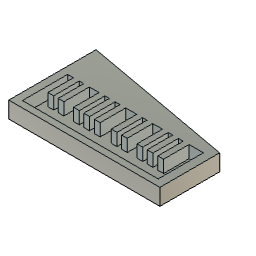
pianoooooo (Autodesk Fusion 360 design; units mm, degrees)
Autodesk Fusion 360 part; units mm, degrees
sketch "草图1" plane through (0, 0, 0) normal (0, 0, 1) x (1, 0, 0)
  line L0 (-83.7376, 48.3346) -> (-83.7376, -57.8018)
  line L1 (100, -57.8018) -> (-83.7376, -57.8018)
  line L2 (99.9425, 14.822) -> (-83.7376, 48.3346)
  line L3 (99.9425, 14.822) -> (99.9425, -57.8018)
  line L4 (-75.3044, 2.9706) -> (90.6956, 2.9706)
  line L5 (90.6956, 2.9706) -> (90.6956, -51.4889)
  line L6 (90.6956, -51.4889) -> (-75.3044, -51.4889)
  line L7 (-75.3044, -51.4889) -> (-75.3044, 2.9706)
  dimension "d1" = 166
  constraint vertical L0
  constraint perpendicular L0 L1
  constraint vertical L3
  constraint horizontal L4
  constraint vertical L5
  constraint horizontal L6
  constraint vertical L7
  measures "d1" distance of L4.start L4.end
extrude "拉伸1" add sketch "草图1" along normal blind 20 contours L0 L1 L2 L3 | L4 L5 L6 L7
sketch "草图2" plane through (0, 0, 20) normal (0, 0, 1) x (-1, 0, 0)
  line L0 (83.7376, -48.3346) -> (83.7376, 57.8018)
  line L1 (83.7376, 57.8018) -> (-99.9425, 57.8018)
  line L2 (-99.9425, 57.8018) -> (-99.9425, -14.822)
  line L3 (-99.9425, -14.822) -> (83.7376, -48.3346)
  line L4 (75, -5) -> (-90, -5)
  line L5 (-90, -5) -> (-90, 50)
  line L6 (-90, 50) -> (75, 50)
  line L7 (75, 50) -> (75, -5)
  constraint horizontal L4
  constraint vertical L5
  constraint horizontal L6
  constraint vertical L7
extrude "拉伸2" cut sketch "草图2" against normal blind 15 contours L4 L5 L6 L7
sketch "草图3" plane through (0, 0, 20) normal (0, 0, 1) x (-1, 0, 0)
  line L0 (-90, -5) -> (-90, 50)
  line L1 (-90, 50) -> (75, 50)
  line L2 (75, 50) -> (75, -5)
  line L3 (75, -5) -> (-90, -5)
  line L4 (83.7376, -48.3346) -> (83.7376, 57.8018)
  line L5 (83.7376, 57.8018) -> (-99.9425, 57.8018)
  line L6 (-99.9425, 57.8018) -> (-99.9425, -14.822)
  line L7 (-99.9425, -14.822) -> (83.7376, -48.3346)
  line L8 (67.985, -5) -> (60.985, -5)
  line L9 (60.985, -5) -> (60.985, 26)
  line L10 (60.985, 26) -> (67.985, 26)
  line L11 (67.985, 26) -> (67.985, -5)
  line L12 (67.985, -5) -> (60.985, -5)
  line L13 (67.985, 26) -> (67.985, -5)
  line L14 (60.985, 26) -> (67.985, 26)
  line L15 (60.985, -5) -> (60.985, 26)
  line L16 (55.5549, 26) -> (55.5549, -5)
  line L17 (55.5549, -5) -> (48.5549, -5)
  line L18 (48.5549, -5) -> (48.5549, 26)
  line L19 (48.5549, 26) -> (55.5549, 26)
  line L20 (55.5549, 26) -> (55.5549, -5)
  line L21 (48.5549, 26) -> (55.5549, 26)
  line L22 (48.5549, -5) -> (48.5549, 26)
  line L23 (55.5549, -5) -> (48.5549, -5)
  line L24 (36.7829, -5) -> (29.7829, -5)
  line L25 (36.7829, 26) -> (36.7829, -5)
  line L26 (29.7829, 26) -> (36.7829, 26)
  line L27 (29.7829, -5) -> (29.7829, 26)
  line L28 (24.3528, 26) -> (24.3528, -5)
  line L29 (17.3528, 26) -> (24.3528, 26)
  line L30 (17.3528, -5) -> (17.3528, 26)
  line L31 (24.3528, -5) -> (17.3528, -5)
  line L32 (11.4154, 26) -> (11.4154, -5)
  line L33 (4.4154, -5) -> (4.4154, 26)
  line L34 (11.4154, -5) -> (4.4154, -5)
  line L35 (4.4154, 26) -> (11.4154, 26)
  line L36 (-52.6472, -5) -> (-59.6472, -5)
  line L37 (-21.4451, 26) -> (-21.4451, -5)
  line L38 (-9.015, -5) -> (-16.015, -5)
  line L39 (-28.4451, 26) -> (-21.4451, 26)
  line L40 (-28.4451, 26) -> (-21.4451, 26)
  line L41 (-40.2171, 26) -> (-40.2171, -5)
  line L42 (-40.2171, -5) -> (-47.2171, -5)
  line L43 (-72.5846, -5) -> (-72.5846, 26)
  line L44 (-47.2171, 26) -> (-40.2171, 26)
  line L45 (-47.2171, -5) -> (-47.2171, 26)
  line L46 (-52.6472, 26) -> (-52.6472, -5)
  line L47 (-65.5846, 26) -> (-65.5846, -5)
  line L48 (-9.015, 26) -> (-9.015, -5)
  line L49 (-16.015, 26) -> (-9.015, 26)
  line L50 (-21.4451, -5) -> (-28.4451, -5)
  line L51 (-28.4451, -5) -> (-28.4451, 26)
  line L52 (-16.015, -5) -> (-16.015, 26)
  line L53 (-28.4451, -5) -> (-28.4451, 26)
  line L54 (-9.015, -5) -> (-16.015, -5)
  line L55 (-16.015, 26) -> (-9.015, 26)
  line L56 (-72.5846, 26) -> (-65.5846, 26)
  line L57 (-65.5846, -5) -> (-72.5846, -5)
  line L58 (-21.4451, 26) -> (-21.4451, -5)
  line L59 (-9.015, 26) -> (-9.015, -5)
  line L60 (-21.4451, -5) -> (-28.4451, -5)
  line L61 (-59.6472, 26) -> (-52.6472, 26)
  line L62 (-59.6472, -5) -> (-59.6472, 26)
  line L63 (-16.015, -5) -> (-16.015, 26)
  line L64 (-82.7432, 26.3749) -> (-82.7432, -4.6251)
  line L65 (-89.7432, 26.3749) -> (-82.7432, 26.3749)
  line L66 (-89.7432, -4.6251) -> (-89.7432, 26.3749)
  line L67 (-82.9307, -4.8125) -> (-89.9307, -4.8125)
  point P0 (-77, 0)
  dimension "d6" = 7
  dimension "d7" = 31
  dimension "d8" = 7
  dimension "d9" = 31
  dimension "d10" = 7
  dimension "d11" = 31
  dimension "d12" = 7
  dimension "d13" = 31
  dimension "d14" = 7
  dimension "d15" = 31
  dimension "d16" = 31
  dimension "d17" = 7
  dimension "d18" = 31
  dimension "d19" = 7
  dimension "d22" = -77
  dimension "d23" = 0
  dimension "d24" = 7
  dimension "d25" = 31
  dimension "d26" = 7
  constraint horizontal L8
  constraint vertical L9
  constraint horizontal L10
  constraint vertical L11
  constraint coincident L3 L8.start
  constraint horizontal L12
  constraint vertical L15
  constraint horizontal L14
  constraint vertical L13
  constraint horizontal L17
  constraint vertical L18
  constraint horizontal L19
  constraint vertical L16
  constraint horizontal L23
  constraint vertical L22
  constraint horizontal L21
  constraint vertical L20
  constraint horizontal L24
  constraint vertical L27
  constraint horizontal L26
  constraint vertical L25
  constraint horizontal L29
  constraint vertical L28
  constraint horizontal L31
  constraint vertical L30
  constraint horizontal L35
  constraint vertical L32
  constraint horizontal L34
  constraint vertical L33
  constraint vertical L66
  constraint horizontal L65
  constraint vertical L64
  constraint horizontal L67
  measures "d6" distance of L8.start L8.end
  measures "d7" distance of L8.start L10.end
  measures "d8" distance of L8.start L8.end
  measures "d9" distance of L8.start L10.end
  measures "d10" distance of L17.end L16.end
  measures "d11" distance of L16.start L16.end
  measures "d12" distance of L17.end L16.end
  measures "d13" distance of L16.start L16.end
  measures "d14" distance of L24.start L24.end
  measures "d15" distance of L25.start L24.start
  measures "d16" distance of L28.end L28.start
  measures "d17" distance of L30.start L28.end
  measures "d18" distance of L32.end L32.start
  measures "d19" distance of L32.end L33.start
  measures "d24" distance of L64.end L66.start
  measures "d25" distance of L64.end L64.start
  measures "d26" distance of L67.end L67.start
extrude "拉伸3" add sketch "草图3" against normal blind 15 contours L3 L43 L47 L56 L57 | L3 L36 L46 L61 L62 | L3 L8 L9 L10 L11 L12 L13 L14 L15 | L3 L41 L42 L44 L45 | L3 L16 L17 L18 L19 L20 L21 L22 L23 | L3 L37 L39 L40 L50 L51 L53 L58 L60 | L3 L24 L25 L26 L27 | L3 L38 L48 L49 L52 L54 L55 L59 L63 | L3 L28 L29 L30 L31 | L3 L32 L33 L34 L35
sketch "草图4" plane through (0, 0, 20) normal (0, 0, 1) x (-1, 0, 0)
  line L0 (-90, -5) -> (-90, 50)
  line L1 (-90, 50) -> (75, 50)
  line L2 (75, 50) -> (75, -5)
  line L3 (75, -5) -> (67.985, -5)
  line L4 (67.985, -5) -> (67.985, 26)
  line L5 (67.985, 26) -> (60.985, 26)
  line L6 (60.985, 26) -> (60.985, -5)
  line L7 (60.985, -5) -> (55.5549, -5)
  line L8 (55.5549, -5) -> (55.5549, 26)
  line L9 (55.5549, 26) -> (48.5549, 26)
  line L10 (48.5549, 26) -> (48.5549, -5)
  line L11 (48.5549, -5) -> (36.7829, -5)
  line L12 (36.7829, -5) -> (36.7829, 26)
  line L13 (36.7829, 26) -> (29.7829, 26)
  line L14 (29.7829, 26) -> (29.7829, -5)
  line L15 (29.7829, -5) -> (24.3528, -5)
  line L16 (24.3528, -5) -> (24.3528, 26)
  line L17 (24.3528, 26) -> (17.3528, 26)
  line L18 (17.3528, 26) -> (17.3528, -5)
  line L19 (17.3528, -5) -> (11.4154, -5)
  line L20 (11.4154, -5) -> (11.4154, 26)
  line L21 (11.4154, 26) -> (4.4154, 26)
  line L22 (4.4154, 26) -> (4.4154, -5)
  line L23 (4.4154, -5) -> (-9.015, -5)
  line L24 (-9.015, -5) -> (-9.015, 26)
  line L25 (-9.015, 26) -> (-16.015, 26)
  line L26 (-16.015, 26) -> (-16.015, -5)
  line L27 (-16.015, -5) -> (-21.4451, -5)
  line L28 (-21.4451, -5) -> (-21.4451, 26)
  line L29 (-21.4451, 26) -> (-28.4451, 26)
  line L30 (-28.4451, 26) -> (-28.4451, -5)
  line L31 (-28.4451, -5) -> (-40.2171, -5)
  line L32 (-40.2171, -5) -> (-40.2171, 26)
  line L33 (-40.2171, 26) -> (-47.2171, 26)
  line L34 (-47.2171, 26) -> (-47.2171, -5)
  line L35 (-47.2171, -5) -> (-52.6472, -5)
  line L36 (-52.6472, -5) -> (-52.6472, 26)
  line L37 (-52.6472, 26) -> (-59.6472, 26)
  line L38 (-59.6472, 26) -> (-59.6472, -5)
  line L39 (-59.6472, -5) -> (-65.5846, -5)
  line L40 (-65.5846, -5) -> (-65.5846, 26)
  line L41 (-65.5846, 26) -> (-72.5846, 26)
  line L42 (-72.5846, 26) -> (-72.5846, -5)
  line L43 (-72.5846, -5) -> (-90, -5)
  line L44 (83.7376, -48.3346) -> (83.7376, 57.8018)
  line L45 (83.7376, 57.8018) -> (-99.9425, 57.8018)
  line L46 (-99.9425, 57.8018) -> (-99.9425, -14.822)
  line L47 (-99.9425, -14.822) -> (83.7376, -48.3346)
